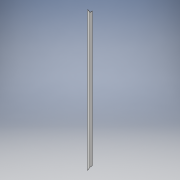
# Autodesk Inventor part: Left_Brace
Saved by Autodesk Inventor 2017 (Build 210142000, 142)
## iProperties
Created: 2018-10-22
Part Number: Left_Brace
Material: Generic
Document SubType Name: Modeling
Designer: mcgratta
Density: 1 g/cm^3
Appearance: Default
Author: mcgratta
Autodesk Inventor part; units mm, degrees
ref_plane "YZ Plane" through (0, 0, 0) normal (1, 0, 0) x (0, 1, 0)
ref_plane "XZ Plane" through (0, 0, 0) normal (0, 1, 0) x (-1, 0, 0)
ref_plane "XY Plane" through (0, 0, 0) normal (0, 0, 1) x (1, 0, 0)
sketch "Sketch1" plane through (0, 0, 0) normal (0, 1, 0) x (-1, 0, 0)
  line L0 (0, 0) -> (38.1, 0)
  line L1 (38.1, 0) -> (38.1, -3.175)
  line L2 (38.1, -3.175) -> (3.175, -3.175)
  line L3 (3.175, -3.175) -> (3.175, -38.1)
  line L4 (3.175, -38.1) -> (0, -38.1)
  line L5 (0, -38.1) -> (0, 0)
  dimension "d0" = 3.175
  dimension "d1" = 3.175
  dimension "d2" = 38.1
  dimension "d3" = 38.1
  constraints: 12 end point, 5 perpendicular, 1 horizontal
  measures "d0" distance between parallel lines of L2 L0
  measures "d1" distance between parallel lines of L5 L3
  measures "d2" distance between parallel lines of L4 L0
  measures "d3" distance between parallel lines of L5 L1
extrude "Extrusion1" add sketch "Sketch1" along normal blind 2133.6
sketch "Sketch2" plane through (0, 0, 0) normal (0, 0, 1) x (1, 0, 0)
  line L0 (0, 0) -> (-38.1, 0) projected
  line L1 (-38.1, 0) -> (0, 0)
  line L2 (0, 0) -> (-38.1, 0)
  line L3 (-38.1, 0) -> (0, 65.9911)
  line L4 (0, 0) -> (0, 2133.6) projected
  line L5 (-38.1, 0) -> (-38.1, 2133.6) projected
  line L6 (-38.1, 2133.6) -> (0, 2111.603)
  line L7 (-38.1, 2133.6) -> (0, 2133.6) projected
  line L8 (0, 2111.603) -> (0, 2133.6)
  line L9 (0, 2133.6) -> (-38.1, 2133.6)
  dimension "d6" = 60
  dimension "d7" = 60
  constraints: 12 end point, 3 collinear, 2 point on line, 1 vertical
  measures "d6" angle of L0 L3
  measures "d7" angle of L4 L6
extrude "Extrusion2" cut sketch "Sketch2" against normal blind 76.2 contours L0 L3 L4
extrude "Extrusion3" cut sketch "Sketch2" against normal blind 76.2 contours L7 L4 L6
body "Solid1"
